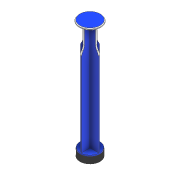
# Autodesk Inventor part: 10 mL syringe plunger
Saved by Autodesk Inventor 2020 (Build 240168000, 168)
## iProperties
Created: 2021-07-28
Part Number: 10 mL syringe plunger
Material: Generic
Document SubType Name: Modeling
Designer: ferrerx
Density: 1 g/cm^3
Appearance: Clear - Blue
Author: ferrerx
Autodesk Inventor part; units mm, degrees
ref_plane "YZ Plane" through (0, 0, 0) normal (1, 0, 0) x (0, 1, 0)
ref_plane "XZ Plane" through (0, 0, 0) normal (0, 1, 0) x (-1, 0, 0)
ref_plane "XY Plane" through (0, 0, 0) normal (0, 0, 1) x (1, 0, 0)
sketch "Sketch1" plane through (0, 0, 0) normal (0, 1, 0) x (-1, 0, 0)
  circle A0 centre (0, 0) radius 7.5
  dimension "d0" = 15
  constraints: 1 centre point, 1 coincident
  measures "d0" diameter of A0
extrude "Extrusion1" add sketch "Sketch1" along normal blind 1
sketch "Sketch2" plane through (0, 1, 0) normal (0, 1, 0) x (1, 0, 0)
  line L0 (-0.565, -6.85) -> (0.565, -6.85)
  line L1 (0.565, -6.85) -> (0.565, 6.85)
  line L2 (0.565, 6.85) -> (-0.565, 6.85)
  line L3 (-0.565, 6.85) -> (-0.565, -6.85)
  line L4 (-0.565, -6.85) -> (0.565, 6.85) construction
  line L5 (0.565, -6.85) -> (-0.565, 6.85) construction
  line L6 (6.85, -0.565) -> (-6.85, -0.565)
  line L7 (-6.85, -0.565) -> (-6.85, 0.565)
  line L8 (-6.85, 0.565) -> (6.85, 0.565)
  line L9 (6.85, 0.565) -> (6.85, -0.565)
  line L10 (6.85, -0.565) -> (-6.85, 0.565) construction
  line L11 (-6.85, -0.565) -> (6.85, 0.565) construction
  point P0 (0, 0)
  point P1 (0.565, 0.565)
  point P2 (-0.565, 0.565)
  point P3 (-0.565, -0.565)
  point P4 (0.565, -0.565)
  dimension "d3" = 13.7
  dimension "d4" = 13.7
  dimension "d5" = 1.13
  dimension "d6" = 1.13
  constraints: 24 end point, 4 midpoint, 4 parallel, 2 horizontal, 2 perpendicular
  measures "d3" distance of L0.end L1.end
  measures "d4" distance of L7.end L8.end
  measures "d5" distance of L1.end L2.end
  measures "d6" distance of L6.end L7.end
extrude "Extrusion2" add sketch "Sketch2" along normal blind 83.3
sketch "Sketch3" plane through (0, 84.3, 0) normal (0, 1, 0) x (1, 0, 0)
  circle A0 centre (0, 0) radius 8.25
  dimension "d9" = 16.5
  constraints: 1 centre point, 1 coincident
  measures "d9" diameter of A0
extrude "Extrusion3" add sketch "Sketch3" along normal blind 1.5
sketch "Sketch4" plane through (6.85, 1, -0.565) normal (1, 0, 0) x (0, 0, -1)
  line L0 (-1.13, 0) -> (-1.13, 83.3) projected
  line L1 (0, 0) -> (0, 83.3) projected
  line L2 (-1.13, 83.3) -> (0, 83.3)
  line L3 (0, 83.3) -> (0, 66.3)
  line L4 (0, 66.3) -> (-1.13, 66.3)
  line L5 (-1.13, 66.3) -> (-1.13, 83.3)
  point P0 (-0.565, -1)
  dimension "d12" = 17
  constraints: 8 end point, 2 parallel, 1 horizontal, 1 perpendicular, 1 point on line
  measures "d12" distance between parallel lines of L4 L2
extrude "Extrusion4" cut sketch "Sketch4" against normal blind 2
pattern_circular "Circular Pattern1" count 4 over 360 about axis through (0, 84.3, 0) along (0, 1, 0) of "Extrusion4"
fillet "Fillet1" radius 5 8 edges at (4.85, 67.3, 0) (0, 67.3, -4.85) (-4.85, 67.3, 0) (0, 67.3, 4.85) (-6.85, 67.3, 0) (0, 67.3, 6.85) (0, 67.3, -6.85) (6.85, 67.3, 0)
fillet "Fillet2" radius 2 4 edges at (0, 84.3, -4.85) (-4.85, 84.3, 0) (0, 84.3, 4.85) (4.85, 84.3, 0)
fillet "Fillet3" radius 0.5 2 edges at (-8.25, 84.3, 0) (-8.25, 85.8, 0)
sketch "Sketch6" plane through (0, 0, 0) normal (0, 0, 1) x (1, 0, 0)
  line L0 (-7.7, 0) -> (-7.7, -4.8)
  line L1 (-7.7, -4.8) -> (0, -7.8)
  line L2 (0, -7.8) -> (0, 0)
  line L3 (0, 0) -> (-7.7, 0)
  line L4 (0, -26.52) -> (0, 104.52) projected
  dimension "d22" = 4.8
  dimension "d23" = 7.7
  dimension "d24" = 3
  constraints: 8 end point, 1 parallel, 1 perpendicular, 1 vertical
  measures "d22" distance of L0.start L0.end
  measures "d23" distance of L2.end L0.start
  measures "d24" vertical distance of L0.end L1.end
revolve "Revolution1" add sketch "Sketch6" angle 360 about axis through (0, 0, 0) along (0, 1, 0)
body "Solid1"
